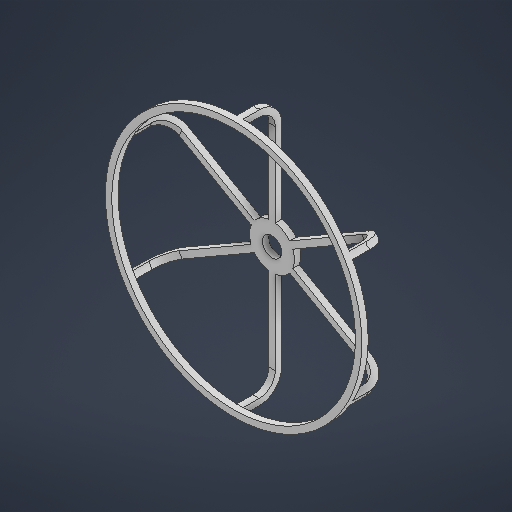
# Autodesk Inventor part: blade_guard
Saved by Autodesk Inventor 2026 (Build 300175050, 175E)
## iProperties
Created: 2025-09-19
Part Number: blade_guard
Material: 일반
Document SubType Name: Modeling
Designer: ytw32
Density: 1 g/cm^3
Appearance: 기본값
Author: ytw32
Autodesk Inventor part; units mm, degrees
ref_plane "YZ Plane" through (0, 0, 0) normal (1, 0, 0) x (0, 1, 0)
ref_plane "XZ Plane" through (0, 0, 0) normal (0, 1, 0) x (-1, 0, 0)
sketch "스케치1" plane through (0, 0, 0) normal (0, 0, 1) x (1, 0, 0)
  circle A0 centre (0, 0) radius 15
  circle A1 centre (0, 0) radius 35
  dimension "d0" = 30
  dimension "d1" = 70
  constraints: 2 centre point, 2 coincident
  measures "d0" diameter of A0
  measures "d1" diameter of A1
extrude "돌출1" add sketch "스케치1" along normal blind 10
sketch "스케치2" plane through (0, 0, 0) normal (1, 0, 0) x (0, 1, 0)
  line L0 (0, 0) -> (190, 0)
  line L1 (190, 0) -> (190, 60)
  line L2 (35, 0) -> (35, 10) projected
  line L3 (35, 0) -> (165, 0)
  line L4 (190, 60) -> (200, 60)
  line L5 (165, 0) -> (165, 35)
  line L6 (165, 0) -> (165, 10)
  arc A0 (165, 10) -> (190, 35) centre (165, 35) ccw
  arc A1 (165, 0) -> (200, 35) centre (165, 35) ccw
  line L7 (200, 60) -> (200, 35)
  line L8 (165, 10) -> (35, 10)
  line L9 (35, 10) -> (25, 10)
  line L10 (35, 10) -> (-35, 10) projected
  line L11 (25, 10) -> (25, 0)
  dimension "d4" = 190
  dimension "d5" = 60
  dimension "d6" = 130
  dimension "d7" = 10
  dimension "d8" = 35
  dimension "d9" = 10
  dimension "d15" = 10
  constraints: 20 end point, 7 point on line, 4 point on circle, 2 centre point, 2 coincident, 2 horizontal, 2 perpendicular, 2 vertical
  measures "d4" distance of L0.start L0.end
  measures "d5" distance of L0.end L1.end
  measures "d6" distance of L3.start L3.end
  measures "d7" distance of L1.end L4.end
  measures "d8" distance of L3.end L5.end
  measures "d9" distance of L3.end L6.end
  measures "d15" distance of L2.end L9.end
extrude "돌출2" add sketch "스케치2" along normal mid plane 10 contours L11 L9 L2 L0 | L2 L8 L5 L0 | L5 A0 L1 A1 | L1 L4 L7 A1
pattern_circular "원형 패턴1" count 6 over 360 about axis through (0, 0, -10) along (0, 0, 1) of "돌출2"
ref_plane "작업 평면1" through (0, 0, 60) normal (0, 0, 1) x (1, 0, 0)
sketch "스케치3" plane through (0, 0, 60) normal (0, 0, 1) x (1, 0, 0)
  circle A0 centre (0, 0) radius 15 projected
  circle A1 centre (0, 0) radius 190
  circle A2 centre (0, 0) radius 200
  circle A3 centre (0, 0) radius 220
  dimension "d17" = 440
  constraints: 3 centre point, 3 coincident
  measures "d17" diameter of A3
extrude "돌출3" add sketch "스케치3" along normal blind 10 contours A2
extrude "돌출4" cut sketch "스케치3" against normal blind 70 contours A3
